stock v1 (Autodesk Fusion 360 design; units mm, degrees)
Autodesk Fusion 360 part; units mm, degrees
box "BoxPrimitive1" add length 300 width 300 height 25 placed x (0, 0, 1) y (1, 0, 0) z (0, 1, 0) at (0, 0, 0)
sketch "Sketch2" plane through (0, 25, 0) normal (0, 1, 0) x (-1, 0, 0)
  line L0 (0, 300) -> (-300, 300)
  line L1 (-300, 300) -> (-300, 0)
  line L2 (-300, 0) -> (0, 0)
  line L3 (0, 0) -> (0, 300)
  line L4 (0, 0) -> (-300, 300)
  line L5 (0, 300) -> (-300, 0)
  line L6 (-150, 150) -> (-300, 150)
  line L7 (-150, 150) -> (0, 150)
  constraint coincident L2.end L3.start
  constraint coincident L0.end L1.start
  constraint coincident L0.start L3.end
  constraint coincident L1.end L2.start
  constraint midpoint L4 L6.start
  constraint midpoint L1 L6.end
  constraint midpoint L3 L7.end
sketch "Sketch3" plane through (0, 25, 0) normal (0, 1, 0) x (-1, 0, 0)
  line L0 (-300, 146.95) -> (0, 146.95)
  line L1 (0, 146.95) -> (0, 153.05)
  line L2 (0, 153.05) -> (-300, 153.05)
  line L3 (-300, 153.05) -> (-300, 146.95)
  line L4 (-300, 146.95) -> (0, 153.05) construction
  line L5 (0, 146.95) -> (-300, 153.05) construction
  point P0 (-150, 150)
  point P1 (-150, 150)
  dimension "d6" = 6.1
  constraint horizontal L0
  constraint perpendicular L0 L1
  constraint parallel L0 L2
  constraint parallel L1 L3
  constraint coincident L4 P1
  constraint coincident L5 P1
  constraint coincident P1 P0
  measures "d6" distance of L0.end L1.end
extrude "Extrude1" cut sketch "Sketch3" against normal blind 24
